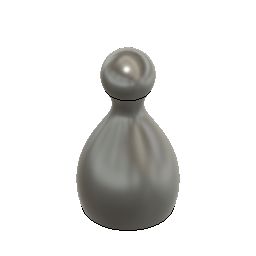
Clobrdo (Autodesk Fusion 360 design; units mm, degrees)
Autodesk Fusion 360 part; units mm, degrees
note: some values were not read from the file. Set by a fixed rule: which sketch regions a step uses.
sketch "Sketch1" plane through (0, 0, 0) normal (0, 0, 1) x (1, 0, 0)
  line L0 (-2.5, 0) -> (-7.5, 0)
  line L1 (0, 2.9) -> (0, 30)
  circle A0 centre (0, 25.5) radius 4.5
  spline S0 degree 5 poles (-7.5, 0) (-7.6079, 0.3272) (-7.8067, 0.9788) (-8.0535, 1.9473) (-8.2798, 3.2212) (-8.3897, 4.7833) (-8.3273, 6.313) (-8.0966, 7.8065) (-7.7081, 9.2577) (-7.1806, 10.6586) (-6.5449, 11.9976) (-5.8419, 13.2617) (-5.1176, 14.4391) (-4.4192, 15.5214) (-3.7912, 16.5064) (-3.2705, 17.4012) (-2.8827, 18.2249) (-2.6432, 19.0042) (-2.5596, 19.7672) (-2.6325, 20.5391) (-2.8577, 21.3361) (-3.1543, 22.0012) (-3.4395, 22.5173) (-3.657, 22.8692) (-3.7727, 23.0471) knots 0 0 0 0 0 0 0.05 0.1 0.15 0.2 0.25 0.3 0.35 0.4 0.45 0.5 0.55 0.6 0.65 0.7 0.75 0.8 0.85 0.9 0.95 1 1 1 1 1 1
  line L2 (-2.5, 0) -> (-2.5, 2.9)
  line L3 (-2.5, 2.9) -> (0, 2.9)
  point P0 (-7.5, 9.7567)
  point P1 (-3.7796, 16.5473)
  point P2 (-2.5986, 19.795)
  dimension "d2" = 30
  dimension "d3" = 9
  dimension "d5" = 2.9
  dimension "d7" = 7.5
  dimension "d8" = 2.5
  constraint horizontal L0
  constraint perpendicular L0 L1
  constraint coincident L1 A0.centre
  constraint coincident L1.end A0
  constraint coincident A0 S0.end
  constraint tangent A0 S0
  constraint perpendicular L0 L2
  constraint perpendicular L2 L3
  constraint vertical origin A0.centre
  constraint horizontal origin L0.start
  measures "d2" distance of origin L1.end
  measures "d3" diameter of A0
  measures "d5" distance of L0.start L2.end
  measures "d7" distance of L0.end L1
  measures "d8" distance of L2.end L1.start
revolve "Revolve1" add sketch "Sketch1" angle 360 about axis through (0, 2.9, 0) along (0, 1, 0) contours L0 L1 A0 S0 L2 L3 | L1 A0 picked at (-2.2746, 26.0368)
chamfer "Chamfer1" distance 0.2 angle 45 1 edges at (-2.3308, 0, 0.904)
named bodies: "Clobrdo"
